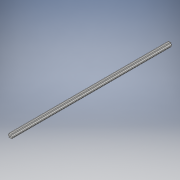
# Autodesk Inventor part: Outtake_churro
Saved by Autodesk Inventor 2018 (Build 220112000, 112)
## iProperties
Created: 2018-09-10
Part Number: Outtake_churro
Material: Generic
Document SubType Name: Modeling
Designer: baoan
Density: 1 g/cm^3
Appearance: Default
Author: baoan
Autodesk Inventor part; units mm, degrees
ref_plane "YZ Plane" through (0, 0, 0) normal (1, 0, 0) x (0, 1, 0)
ref_plane "XZ Plane" through (0, 0, 0) normal (0, 1, 0) x (-1, 0, 0)
ref_plane "XY Plane" through (0, 0, 0) normal (0, 0, 1) x (1, 0, 0)
sketch "Sketch1" plane through (0, 0, 0) normal (0, 0, 1) x (1, 0, 0)
  line L0 (-3.6662, 6.35) -> (-1.8331, 6.35)
  line L1 (3.6662, 6.35) -> (4.5827, 4.7625)
  line L2 (7.3323, 0) -> (6.4158, -1.5875)
  line L3 (3.6662, -6.35) -> (1.8331, -6.35)
  line L4 (-3.6662, -6.35) -> (-4.5827, -4.7625)
  line L5 (-7.3323, 0) -> (-6.4158, 1.5875)
  arc A0 (-1.8331, 6.35) -> (1.8331, 6.35) centre (0, 6.35) ccw
  arc A1 (-6.4158, 1.5875) -> (-4.5827, 4.7625) centre (-5.4993, 3.175) ccw
  arc A2 (-4.5827, -4.7625) -> (-6.4158, -1.5875) centre (-5.4993, -3.175) ccw
  arc A3 (1.8331, -6.35) -> (-1.8331, -6.35) centre (0, -6.35) ccw
  arc A4 (6.4158, -1.5875) -> (4.5827, -4.7625) centre (5.4993, -3.175) ccw
  arc A5 (4.5827, 4.7625) -> (6.4158, 1.5875) centre (5.4993, 3.175) ccw
  line L6 (-1.8331, 6.35) -> (1.8331, 6.35) construction
  line L7 (1.8331, 6.35) -> (3.6662, 6.35)
  line L8 (-4.5827, 4.7625) -> (-3.6662, 6.35)
  line L9 (-6.4158, 1.5875) -> (-4.5827, 4.7625) construction
  line L10 (-4.5827, -4.7625) -> (-6.4158, -1.5875) construction
  line L11 (-6.4158, -1.5875) -> (-7.3323, 0)
  line L12 (-1.8331, -6.35) -> (-3.6662, -6.35)
  line L13 (1.8331, -6.35) -> (-1.8331, -6.35) construction
  line L14 (4.5827, -4.7625) -> (3.6662, -6.35)
  line L15 (6.4158, -1.5875) -> (4.5827, -4.7625) construction
  line L16 (6.4158, 1.5875) -> (7.3323, 0)
  line L17 (4.5827, 4.7625) -> (6.4158, 1.5875) construction
  circle A6 centre (0, 0) radius 2.0701
  dimension "d0" = 12.7
  dimension "d1" = 1.8331
  dimension "d4" = 360
  dimension "d6" = 1.8331
  dimension "d7" = 1.8331
  dimension "d8" = 4.1402
  constraints: 36 end point, 12 point on circle, 7 centre point, 3 horizontal, 2 coincident, 1 point on line, 38 other
  measures "d0" distance between parallel lines of L3 L0
  measures "d1" radius of A0
  measures "d6" distance of L1.start L6.end
  measures "d7" distance of L0.start L0.end
  measures "d8" diameter of A6
extrude "Extrusion1" add sketch "Sketch1" along normal mid plane 508
body "Solid1"
